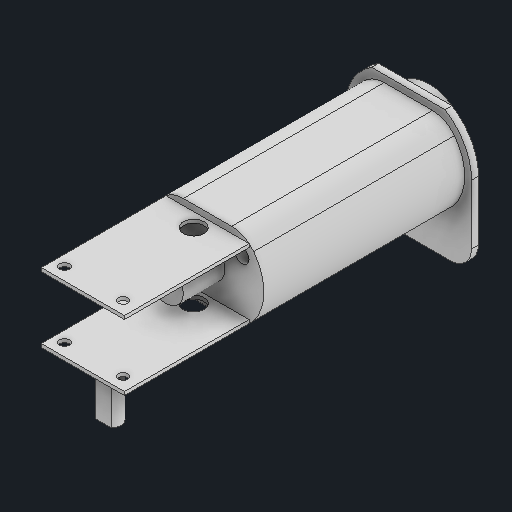
# Autodesk Inventor part: 电机
Saved by Autodesk Inventor 2025 (Build 290162000, 162)
## iProperties
Created: 2025-12-07
Part Number: 电机
Material: 常规
Document SubType Name: Modeling
Designer: XH
Density: 1 g/cm^3
Appearance: 默认
Author: XH
Autodesk Inventor part; units mm, degrees
ref_plane "YZ Plane" through (0, 0, 0) normal (1, 0, 0) x (0, 1, 0)
ref_plane "XZ Plane" through (0, 0, 0) normal (0, 1, 0) x (-1, 0, 0)
ref_plane "XY Plane" through (0, 0, 0) normal (0, 0, 1) x (1, 0, 0)
sketch "草图1" plane through (0, 0, 0) normal (0, 0, 1) x (1, 0, 0)
  line L0 (-5, 0) -> (5, 0) construction
  line L1 (-5, -6.3307) -> (5, -6.3307)
  line L2 (5, 5.4693) -> (-5, 5.4693)
  arc A0 (-5, 5.4693) -> (-5, -6.3307) centre (-1.0059, -0.4307) ccw
  line L3 (0, 0) -> (0, 3.0217)
  arc A1 (5, -6.3307) -> (5, 5.4693) centre (1.0059, -0.4307) ccw
  line L4 (5, 5.4693) -> (5, -6.3307)
  line L5 (-5, 5.4693) -> (-5, -6.3307)
  point P0 (-10.9, 0)
  point P1 (10.9, 0)
  point P2 (10.9, 0)
  dimension "d0" = 11.8
  dimension "d6" = 10
  constraints: 14 end point, 4 point on circle, 2 centre point, 2 perpendicular, 2 symmetric about line, 1 coincident, 1 horizontal, 1 midpoint, 1 parallel, 1 vertical, 1 other
  measures "d0" distance between parallel lines of L1 L2
  measures "d6" distance of L2.start L2.end
extrude "拉伸1" add sketch "草图1" along normal blind 29
sketch "草图2" plane through (0, 0, 29) normal (0, 0, 1) x (1, 0, 0)
  line L0 (6, -5.4307) -> (-6, -5.4307)
  line L1 (-6, -5.4307) -> (-6, 4.5693)
  line L2 (-6, 4.5693) -> (6, 4.5693)
  line L3 (6, 4.5693) -> (6, -5.4307)
  line L4 (6, -5.4307) -> (-6, 4.5693) construction
  line L5 (-6, -5.4307) -> (6, 4.5693) construction
  line L6 (5, 5.4693) -> (-5, 5.4693) projected
  line L7 (0, 5.4693) -> (0, -6.3307)
  line L8 (-5, -6.3307) -> (5, -6.3307) projected
  point P0 (0, -0.4307)
  dimension "d4" = 10
  dimension "d5" = 12
  constraints: 14 end point, 5 midpoint, 2 parallel, 1 horizontal, 1 perpendicular
  measures "d4" distance of L2.end L0.start
  measures "d5" distance between parallel lines of L1 L3
extrude "拉伸2" add sketch "草图2" along normal blind 18
sketch "草图3" plane through (0, 0, 0) normal (0, 0, -1) x (-1, 0, 0)
  line L0 (5, -6.3307) -> (-5, -6.3307) projected
  arc A0 (5, -6.3307) -> (5, 5.4693) centre (1.0059, -0.4307) ccw projected
  line L1 (-5, 5.4693) -> (5, 5.4693) projected
  arc A1 (-5, 5.4693) -> (-5, -6.3307) centre (-1.0059, -0.4307) ccw projected
  arc A2 (5.2957, -7.3307) -> (5.2957, 6.4693) centre (1.0059, -0.4307) ccw
  line L2 (5.2957, -7.3307) -> (-5.2957, -7.3307)
  arc A3 (-5.2957, 6.4693) -> (-5.2957, -7.3307) centre (-1.0059, -0.4307) ccw
  line L3 (-5.2957, 6.4693) -> (5.2957, 6.4693)
  line L4 (-9.1307, -0.4307) -> (9.1307, -0.4307)
  line L5 (9.1307, -0.4307) -> (9.1307, -12.0307)
  line L6 (9.1307, -12.0307) -> (-9.1307, -12.0307)
  line L7 (-9.1307, -12.0307) -> (-9.1307, -0.4307)
  point P0 (0, 0)
  dimension "d9" = 1
  dimension "d10" = 18.5
  constraints: 12 end point, 6 point on circle, 2 centre point, 2 parallel, 1 horizontal, 1 perpendicular, 3 other
  measures "d9" radial gap between concentric circles of A0 A2
  measures "d10" distance between parallel lines of L3 L6
extrude "拉伸3" add sketch "草图3" along normal blind 1
sketch "草图4" plane through (0, 0, -1) normal (0, 0, -1) x (-1, 0, 0)
  circle A0 centre (0, 0) radius 5.5587
  constraints: 1 centre point, 1 coincident
extrude "拉伸4" add sketch "草图4" along normal blind 2
sketch "草图5" plane through (-6, -5.4307, 29) normal (0, 1, 0) x (1, 0, 0)
  circle A0 centre (6, -14) radius 1.5
  line L0 (12, -18) -> (0, -18) projected
  point P0 (6, 29)
  dimension "d15" = 4
  dimension "d16" = 3
  constraints: 1 centre point
  measures "d15" distance from line of A0.centre L0
  measures "d16" diameter of A0
extrude "拉伸5" add sketch "草图5" against normal blind 8
sketch "草图7" plane through (0, -13.4307, 43) normal (0, -1, 0) x (1, 0, 0)
  circle A0 centre (0, 0) radius 1.5 projected
  line L0 (-1.118, 1) -> (1.118, 1)
  point P0 (0, -43)
  point P1 (0, 1.5)
  dimension "d19" = 0.5
  constraints: 3 point on circle, 2 end point, 1 horizontal
  measures "d19" distance edge to line of A0 L0
extrude "拉伸6" cut sketch "草图7" against normal up to surface (8 mm away) contours L0 A0 picked at (-0.0599, 1.1631)
fillet "圆角1" radius 4 4 edges at (-5, 5.4693, 14.5) (5, 5.4693, 14.5) (-5, -6.3307, 14.5) (5, -6.3307, 14.5)
fillet "圆角2" radius 3 2 edges at (-9.1307, -12.0307, -0.5) (9.1307, -12.0307, -0.5)
sketch "草图8" plane through (-6, -5.4307, 29) normal (0, -1, 0) x (1, 0, 0)
  circle A0 centre (10.0294, 16.2) radius 0.7
  circle A1 centre (1.5294, 16.2) radius 0.7
  line L0 (0, 18) -> (12, 18) projected
  point P0 (6, -29)
  dimension "d24" = 1.4
  dimension "d25" = 1.4
  dimension "d26" = 8.5
  dimension "d27" = 1.8
  constraints: 2 centre point, 1 horizontal alignment
  measures "d24" diameter of A0
  measures "d25" diameter of A1
  measures "d26" distance of A0.centre A1.centre
  measures "d27" distance from line of L0 A1.centre
extrude "拉伸7" cut sketch "草图8" against normal blind 11.75
sketch "草图9" plane through (-6, 4.5693, 29) normal (0, 1, 0) x (1, 0, 0)
  line L0 (6, -14) -> (6, -2)
  circle A0 centre (6, -2) radius 1.5
  arc A1 (8.5, -14) -> (3.5, -14) centre (6, -14) ccw projected
  point P0 (6, 29)
  dimension "d30" = 12
  dimension "d31" = 3
  constraints: 2 end point, 1 centre point, 1 coincident, 1 vertical
  measures "d30" distance of L0.start L0.end
  measures "d31" diameter of A0
extrude "拉伸8" cut sketch "草图9" against normal blind 23
sketch "草图10" plane through (0, 0, 29) normal (0, 0, 1) x (1, 0, 0)
  line L0 (-6, 4.5693) -> (6, 4.5693) projected
  line L1 (0, 4.5693) -> (0, -5.4307)
  line L2 (6, -5.4307) -> (-6, -5.4307) projected
  line L3 (8.5655, -4.9307) -> (-8.5655, -4.9307)
  line L4 (-8.5655, -4.9307) -> (-8.5655, 4.0693)
  line L5 (-8.5655, 4.0693) -> (8.5655, 4.0693)
  line L6 (8.5655, 4.0693) -> (8.5655, -4.9307)
  line L7 (8.5655, -4.9307) -> (-8.5655, 4.0693) construction
  line L8 (-8.5655, -4.9307) -> (8.5655, 4.0693) construction
  point P0 (0, 0)
  point P1 (0, -0.4307)
  dimension "d34" = 0.5
  constraints: 14 end point, 5 midpoint, 2 parallel, 1 horizontal, 1 perpendicular
  measures "d34" distance between parallel lines of L0 L5
extrude "拉伸9" cut sketch "草图10" along normal blind 39.5
sketch "草图11" plane through (0, 0, 29) normal (0, 0, 1) x (1, 0, 0)
  circle A0 centre (0, -0.4307) radius 2.5
  arc A1 (-6.6623, 3.9014) -> (-6.6623, -4.7629) centre (-1.0059, -0.4307) ccw projected
  line L0 (-8.1307, -0.4307) -> (8.1307, -0.4307)
  arc A2 (6.6623, -4.7629) -> (6.6623, 3.9014) centre (1.0059, -0.4307) ccw projected
  dimension "d37" = 5
  constraints: 2 end point, 2 point on circle, 1 centre point, 1 coincident, 1 horizontal, 1 midpoint
  measures "d37" diameter of A0
extrude "拉伸10" add sketch "草图11" along normal blind 6
sketch "草图12" plane through (0, 0, 29) normal (0, 0, 1) x (1, 0, 0)
  circle A0 centre (0, -0.4307) radius 5.831
  circle A1 centre (5, 2.5693) radius 1
  circle A2 centre (0, -0.4307) radius 5.5587
  line L0 (0, -0.4307) -> (0, 11.5704)
  line L1 (0, -0.4307) -> (0, 11.9593)
  circle A3 centre (-5, 2.5693) radius 1
  line L2 (0, -0.4307) -> (-7.5185, -0.4307)
  circle A4 centre (-5, -3.4307) radius 1
  arc A5 (-6.6623, 3.9014) -> (-6.6623, -4.7629) centre (-1.0059, -0.4307) ccw projected
  line L3 (-8.1307, -0.4307) -> (8.1307, -0.4307)
  arc A6 (6.6623, -4.7629) -> (6.6623, 3.9014) centre (1.0059, -0.4307) ccw projected
  dimension "d40" = 2
  dimension "d41" = 5
  dimension "d42" = 3
  constraints: 8 end point, 5 centre point, 5 point on circle, 2 horizontal, 2 symmetric about line, 2 vertical, 1 coincident, 1 midpoint, 1 point on line, 2 other
  measures "d40" diameter of A1
  measures "d41" horizontal distance of A1.centre L0.start
  measures "d42" vertical distance of point (0, -0.431) A1.centre
extrude "拉伸11" cut sketch "草图12" against normal blind 6 contours A1 A2 A0 | A0 A1 | A4 A0 | A0 A4 A2 | A1 A2 | A2 A4
